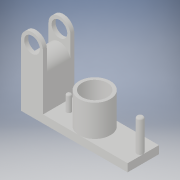
# Autodesk Inventor part: ValveBaseMk2.1
Saved by Autodesk Inventor 2019 (Build 230136000, 136)
## iProperties
Created: 2019-01-19
Part Number: ValveBaseMk2.1
Material: Generic
Document SubType Name: Modeling
Designer: Kepler
Density: 1 g/cm^3
Appearance: Default
Author: Kepler
Autodesk Inventor part; units mm, degrees
ref_plane "YZ Plane" through (0, 0, 0) normal (1, 0, 0) x (0, 1, 0)
ref_plane "XZ Plane" through (0, 0, 0) normal (0, 1, 0) x (-1, 0, 0)
ref_plane "XY Plane" through (0, 0, 0) normal (0, 0, 1) x (1, 0, 0)
sketch "Sketch1" plane through (0, 0, 0) normal (0, 0, 1) x (1, 0, 0)
  line L0 (0, 0) -> (0, 40)
  line L1 (0, 0) -> (68, 0)
  line L2 (68, 0) -> (68, 5)
  line L3 (68, 5) -> (14, 5)
  arc A0 (14, 40) -> (0, 40) centre (7, 40) ccw
  line L4 (14, 40) -> (14, 5)
  circle A1 centre (7, 40) radius 5
  dimension "d0" = 40
  dimension "d2" = 5
  dimension "d6" = 7
  dimension "d7" = 10
  dimension "d8" = 14
  dimension "d9" = 54
  dimension "d46" = 68
  constraints: 10 end point, 3 perpendicular, 2 centre point, 2 point on circle, 2 tangent, 1 coincident, 1 horizontal, 1 vertical
  measures "d0" distance of L0.start L0.end
  measures "d2" distance of L1.end L2.end
  measures "d6" radius of A0
  measures "d7" diameter of A1
  measures "d8" distance between parallel lines of L4 L0
  measures "d9" distance of L2.end L3.end
  measures "d46" distance between parallel lines of L2 L0
extrude "Extrusion1" add sketch "Sketch1" along normal blind 20
sketch "Sketch2" plane through (14, 5, 0) normal (0, 1, 0) x (1, 0, 0)
  circle A0 centre (6.5, -10) radius 1.5
  line L0 (0, 0) -> (0, -20) projected
  circle A1 centre (23, -10) radius 10
  line L1 (0, 0) -> (54, 0) projected
  circle A2 centre (52, -10) radius 2
  line L2 (54, 0) -> (54, -20) projected
  line L3 (-2, 0) -> (-2, -20) projected
  line L4 (-12, 0) -> (-12, -20) projected
  line L5 (-7, -10) -> (-7, -6.6929)
  point P0 (-14, 0)
  dimension "d12" = 3
  dimension "d13" = 6.5
  dimension "d14" = 20
  dimension "d16" = 23
  dimension "d19" = 10
  dimension "d20" = 4
  dimension "d21" = 10
  dimension "d22" = 17
  dimension "d47" = 31
  dimension "d48" = 59
  dimension "d49" = 30
  constraints: 3 centre point, 2 end point, 2 tangent, 1 vertical
  measures "d12" diameter of A0
  measures "d13" distance from line of L0 A0.centre
  measures "d14" diameter of A1
  measures "d16" distance from line of A1.centre L0
  measures "d19" distance from line of L1 A0.centre
  measures "d20" diameter of A2
  measures "d21" distance from line of L1 A2.centre
  measures "d47" distance from line of L2 A1.centre
  measures "d48" distance from line of A2.centre L5
  measures "d49" distance from line of L5 A1.centre
extrude "Extrusion2" add sketch "Sketch2" along normal blind 20
sketch "Sketch4" plane through (0, 0, 20) normal (0, 0, 1) x (1, 0, 0)
  line L0 (22, 25) -> (19, 25) projected
  line L1 (19, 25) -> (22, 25)
  line L2 (22, 5) -> (22, 25) projected
  line L3 (22, 25) -> (22, 15)
  line L4 (22, 15) -> (19, 15)
  line L5 (19, 5) -> (19, 25) projected
  point P0 (0, 0)
  dimension "d25" = 10
  constraints: 6 end point, 2 midpoint, 1 horizontal, 1 point on line
  measures "d25" distance of L1.end L3.end
extrude "Extrusion3" cut sketch "Sketch4" against normal blind 20
fillet "Fillet1" radius 1 1 edges at (19, 15, 10)
fillet "Fillet2" radius 1 1 edges at (64, 25, 10)
sketch "Sketch5" plane through (37, 25, 10) normal (0, 1, 0) x (1, 0, 0)
  circle A0 centre (0, 0) radius 8
  point P0 (-37, 10)
  dimension "d30" = 16
  constraints: 1 centre point
  measures "d30" diameter of A0
extrude "Extrusion4" cut sketch "Sketch5" against normal blind 30
sketch "Sketch6" plane through (14, 5, 0) normal (1, 0, 0) x (0, 0, -1)
  point P0 (0, -5)
sketch "Sketch7" plane through (14, 5, 0) normal (1, 0, 0) x (0, 0, -1)
  line L0 (-10, 41.0364) -> (-10, 39.6436)
  line L1 (0, 42) -> (-20, 42) projected
  line L2 (-2.5, 42) -> (-2.5, 28)
  line L3 (-17.5, 42) -> (-17.5, 28)
  line L4 (-17.5, 42) -> (-2.5, 42)
  line L5 (0, 30) -> (-20, 30) projected
  line L6 (-17.5, 28) -> (-2.5, 28)
  point P0 (0, -5)
  dimension "d12" = 3
  dimension "d40" = 14
  dimension "d41" = 14
  dimension "d42" = 15
  constraints: 10 end point, 2 point on line, 2 vertical, 1 collinear, 1 perpendicular, 1 other
  measures "d40" distance of L2.start L2.end
  measures "d41" distance of L3.start L3.end
  measures "d42" distance between parallel lines of L3 L2
extrude "Extrusion5" cut sketch "Sketch7" against normal blind 14
fillet "Fillet3" radius 7 2 edges at (14, 33, 10) (0, 33, 10)
sketch "Sketch8" plane through (37, 5, 0) normal (0, 1, 0) x (1, 0, 0)
  point P0 (-37, 0)
equation "\"d19\" = 0.5 * d14"
equation "\"d21\" = d19"
equation "\"d40\" = d41"
body "Solid1"
